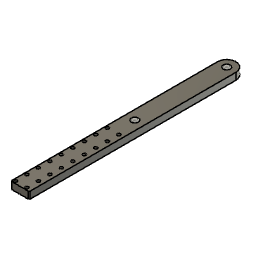
chamber brackets v6 (Autodesk Fusion 360 design; units mm, degrees)
Autodesk Fusion 360 part; units mm, degrees
note: some values were not read from the file. Set by a fixed rule: the direction of a hole.
sketch "Sketch1" plane through (0, 0, 0) normal (0, 1, 0) x (1, 0, 0)
  line L0 (-20, -450) -> (-20, 0)
  arc A0 (20, 0) -> (-20, 0) centre (0, 0) ccw
  line L1 (20, 0) -> (20, -450)
  line L2 (20, -450) -> (-20, -450)
  point P0 (0, -200)
  point P1 (-15, -245)
  dimension "d1" = 20
  dimension "d2" = 450
  dimension "d3" = 200
  dimension "d9" = 45
  dimension "d10" = 15
  constraint vertical L0
  constraint tangent L0 A0
  constraint vertical L1
  constraint horizontal L2
  constraint coincident A0.centre origin
  constraint tangent A0 L1
  constraint vertical A0.centre P0
  measures "d1" radius of A0
  measures "d2" distance of A0.centre L2
  measures "d3" distance of A0.centre P0
  measures "d9" vertical distance of P0 P1
  measures "d10" horizontal distance of P0 P1
extrude "Extrude1" add sketch "Sketch1" along normal blind 15
hole "Hole1" at (0, 0, 200) at (0, 0, 0) direction (0, 1, 0) diameter 15.526 depth 200 tip angle 118
thread "Thread1" "ISO Metric profile 17.0 M17x1.5 6H" thread offset 0 thread depth 10
hole "Hole2" at (-15, 0, 245) direction (0, 1, 0) diameter 7 depth 200 tip angle 118
pattern_linear "R-Pattern1" count 11 spacing 25 along (0, 0, 1) count 2 spacing 25 along (1, 0, 0) of "Hole2"
chamfer "Chamfer1" distance 2 angle 45 2 edges at (20, 7.5, 450) (-20, 7.5, 450)
